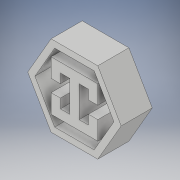
# Autodesk Inventor part: 1
Saved by Autodesk Inventor 2019 (Build 230136000, 136)
## iProperties
Created: 2018-07-31
Part Number: 1
Material: Generic
Document SubType Name: Modeling
Designer: Ge Shi
Density: 1 g/cm^3
Appearance: Default
Author: Ge Shi
Autodesk Inventor part; units mm, degrees
ref_plane "YZ Plane" through (0, 0, 0) normal (1, 0, 0) x (0, 1, 0)
ref_plane "XZ Plane" through (0, 0, 0) normal (0, 1, 0) x (-1, 0, 0)
ref_plane "XY Plane" through (0, 0, 0) normal (0, 0, 1) x (1, 0, 0)
sketch "Sketch1" plane through (0, 0, 0) normal (0, 0, 1) x (1, 0, 0)
  circle A0 centre (0, 0) radius 7.5
  line L0 (-3.75, 6.4952) -> (3.75, 6.4952)
  line L1 (3.75, 6.4952) -> (7.5, 0)
  line L2 (7.5, 0) -> (3.75, -6.4952)
  line L3 (3.75, -6.4952) -> (-3.75, -6.4952)
  line L4 (-3.75, -6.4952) -> (-7.5, 0)
  line L5 (-7.5, 0) -> (-3.75, 6.4952)
  line L6 (-3.1726, 5.4952) -> (3.1726, 5.4952)
  line L7 (3.1726, 5.4952) -> (6.3453, 0)
  line L8 (6.3453, 0) -> (3.1726, -5.4952)
  line L9 (3.1726, -5.4952) -> (-3.1726, -5.4952)
  line L10 (-3.1726, -5.4952) -> (-6.3453, 0)
  line L11 (-6.3453, 0) -> (-3.1726, 5.4952)
  line L12 (0, 3.9952) -> (-3.75, 3.9952)
  line L13 (-3.75, 3.9952) -> (-3.75, 0.9952)
  line L14 (-3.75, 0.9952) -> (-2.25, 0.9952)
  line L15 (-2.25, 0.9952) -> (-2.25, 2.4952)
  line L16 (-2.25, 2.4952) -> (-0.75, 2.4952)
  line L17 (-0.75, 2.4952) -> (-0.75, 0)
  line L18 (-0.75, 0) -> (0, 0)
  line L19 (0, 0) -> (0, 3.9952)
  line L20 (0, 3.9952) -> (3.75, 3.9952)
  line L21 (3.75, 3.9952) -> (3.75, 0.9952)
  line L22 (3.75, 0.9952) -> (2.25, 0.9952)
  line L23 (2.25, 0.9952) -> (2.25, 2.4952)
  line L24 (2.25, 2.4952) -> (0.75, 2.4952)
  line L25 (0.75, 2.4952) -> (0.75, 0)
  line L26 (0.75, 0) -> (0, 0)
  line L27 (0, -3.9952) -> (-3.75, -3.9952)
  line L28 (-3.75, -3.9952) -> (-3.75, -0.9952)
  line L29 (-3.75, -0.9952) -> (-2.25, -0.9952)
  line L30 (-2.25, -0.9952) -> (-2.25, -2.4952)
  line L31 (-2.25, -2.4952) -> (-0.75, -2.4952)
  line L32 (-0.75, -2.4952) -> (-0.75, 0)
  line L33 (2.25, -2.4952) -> (0.75, -2.4952)
  line L34 (0.75, -2.4952) -> (0.75, 0)
  line L35 (3.75, -0.9952) -> (2.25, -0.9952)
  line L36 (2.25, -0.9952) -> (2.25, -2.4952)
  line L37 (3.75, -3.9952) -> (3.75, -0.9952)
  line L38 (0, -3.9952) -> (3.75, -3.9952)
  dimension "d0" = 15
  dimension "d1" = 1
  dimension "d15" = 1.5
  dimension "d16" = 1.5
  dimension "d17" = 1.5
  dimension "d18" = 1.5
  dimension "d19" = 0.75
  dimension "d20" = 1.5
  constraints: 78 end point, 17 symmetric about line, 6 perpendicular, 3 horizontal, 1 vertical, 3 other
  measures "d1" distance between parallel lines of L0 L6
  measures "d15" distance between parallel lines of L13 L15
  measures "d16" distance between parallel lines of L12 L16
  measures "d17" distance between parallel lines of L14 L16
  measures "d18" distance between parallel lines of L6 L12
  measures "d19" distance between parallel lines of L19 L17
  measures "d20" distance between parallel lines of L17 L15
extrude "Extrusion1" add sketch "Sketch1" along normal blind 5 contours L2 L3 L4 L5 L0 L1 | L19 L18 L17 L16 L15 L14 L13 L12 | L20 L21 L22 L23 L24 L25 L26 L19 | L26 L34 L33 L36 L35 L37 L38 L27 L28 L29 L30 L31 L32 L18
body "Solid1"
